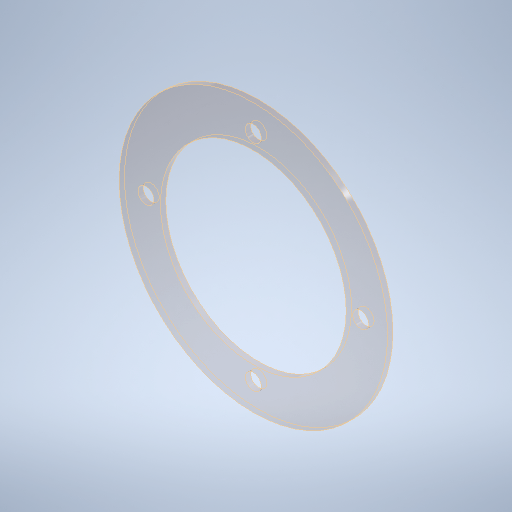
# Autodesk Inventor part: uszczelka
Saved by Autodesk Inventor 2025 (Build 290162000, 162)
## iProperties
Created: 2025-03-23
Part Number: uszczelka
Material: Poliwęglan dymiony
Document SubType Name: Modeling
Designer: barte
Density: 1.2 g/cm^3
Appearance: Poliwęglan — przydymiony
Author: barte
Autodesk Inventor part; units mm, degrees
ref_plane "YZ Plane" through (0, 0, 0) normal (1, 0, 0) x (0, 1, 0)
ref_plane "XZ Plane" through (0, 0, 0) normal (0, 1, 0) x (-1, 0, 0)
ref_plane "XY Plane" through (0, 0, 0) normal (0, 0, 1) x (1, 0, 0)
sketch "Szkic1" plane through (0, 0, 0) normal (0, 1, 0) x (-1, 0, 0)
  line L0 (34.6, 10.4209) -> (34.6, 8.4209)
  line L1 (34.6, 8.4209) -> (50, 8.4209)
  line L2 (50, 8.4209) -> (50, 10.4209)
  line L3 (50, 10.4209) -> (34.6, 10.4209)
  line L4 (0, 0) -> (0, 76.2035)
  dimension "d0" = 15.4
  dimension "d1" = 2
  dimension "d2" = 34.6
  constraints: 10 end point, 2 perpendicular, 2 vertical, 1 horizontal
  measures "d0" distance between parallel lines of L0 L2
  measures "d1" distance between parallel lines of L3 L1
  measures "d2" distance between parallel lines of L4 L0
revolve "Obrót1" add sketch "Szkic1" angle 360 about axis through (0, 0, 0) along (0, 0, 1)
sketch "Szkic5" plane through (0, 0, 10.4209) normal (0, 0, 1) x (1, 0, 0)
  circle A0 centre (0, 40) radius 3
  circle A1 centre (40, 0) radius 3
  circle A2 centre (0, -40) radius 3
  circle A3 centre (-40, 0) radius 3
  point P0 (0, 0)
  dimension "d16" = 6
  dimension "d17" = 6
  dimension "d18" = 6
  dimension "d19" = 6
  constraints: 4 centre point
  measures "d16" diameter of A0
  measures "d17" diameter of A1
  measures "d18" diameter of A2
  measures "d19" diameter of A3
extrude "Wyciągnięcie proste3" cut sketch "Szkic5" against normal blind 2
